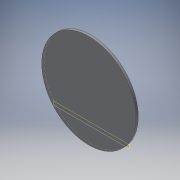
# Autodesk Inventor part: base thingy
Saved by Autodesk Inventor 2019 (Build 230136000, 136)
## iProperties
Created: 2022-03-28
Part Number: base thingy
Material: Generic
Document SubType Name: Modeling
Designer: Ian
Density: 1 g/cm^3
Appearance: Default
Author: Ian
Autodesk Inventor part; units mm, degrees
ref_plane "YZ Plane" through (0, 0, 0) normal (1, 0, 0) x (0, 1, 0)
ref_plane "XZ Plane" through (0, 0, 0) normal (0, 1, 0) x (-1, 0, 0)
ref_plane "XY Plane" through (0, 0, 0) normal (0, 0, 1) x (1, 0, 0)
ref_plane "Work Plane1" through (-150, -140.3395, 0) normal (0, 0, 1) x (-1, 0, 0)
sketch "Sketch1" plane through (-150, -140.3395, 0) normal (0, 0, 1) x (-1, 0, 0)
  circle A0 centre (-75, -70.1697) radius 102.7073
  line L0 (-150, 0) -> (0, 0) projected
  line L1 (-150, 0) -> (-150, -7) projected
  line L2 (0, -7) -> (-150, -7) projected
  line L3 (0, 0) -> (0, -7) projected
  line L4 (0, -140.3395) -> (-150, -140.3395) projected
  line L5 (0, -140.3395) -> (0, -133.3395) projected
  line L6 (-150, -133.3395) -> (0, -133.3395) projected
  line L7 (-150, -140.3395) -> (-150, -133.3395) projected
  line L8 (-75, -70.1697) -> (-75, -172.877)
  line L9 (-75, -70.1697) -> (13.9471, -18.8161)
  line L10 (-75, -70.1697) -> (-163.9471, -18.8161)
  dimension "d0" = 120
  dimension "d1" = 120
  constraints: 6 end point, 6 point on circle, 1 centre point, 1 vertical
  measures "d0" angle of L9 L8
  measures "d1" angle of L10 L8
extrude "Extrusion1" add sketch "Sketch1" along normal blind 5
body "Solid1"
